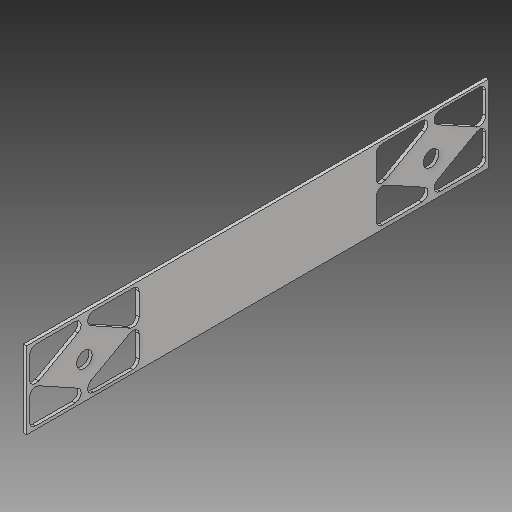
# Autodesk Inventor part: R-SideV1
Saved by Autodesk Inventor 2019 (Build 230136000, 136)
## iProperties
Created: 2021-09-15
Part Number: R-SideV1
Material: Generic
Document SubType Name: Modeling
Designer: timmy
Density: 1 g/cm^3
Appearance: Default
Author: timmy
Autodesk Inventor part; units mm, degrees
ref_plane "YZ Plane" through (0, 0, 0) normal (1, 0, 0) x (0, 1, 0)
ref_plane "XZ Plane" through (0, 0, 0) normal (0, 1, 0) x (-1, 0, 0)
ref_plane "XY Plane" through (0, 0, 0) normal (0, 0, 1) x (1, 0, 0)
sketch "Sketch1" plane through (0, 0, 0) normal (1, 0, 0) x (0, 1, 0)
  line L0 (0, 0) -> (152.4, 0)
  line L1 (152.4, 0) -> (152.4, -914.4)
  line L2 (152.4, -914.4) -> (0, -914.4)
  line L3 (0, -914.4) -> (0, 0)
  dimension "d0" = 152.4
  dimension "d1" = 914.4
  constraints: 8 end point, 2 parallel, 1 horizontal, 1 perpendicular
  measures "d0" distance of L1.end L2.end
  measures "d1" distance of L0.end L1.end
extrude "Extrusion1" add sketch "Sketch1" along normal blind 6.35
sketch "Sketch2" plane through (6.35, 0, 0) normal (1, 0, 0) x (0, 0, -1)
  line L0 (0, 152.4) -> (0, 0) construction
  line L1 (914.4, 152.4) -> (0, 152.4) construction
  line L2 (0, 152.4) -> (457.2, 152.4) construction
  line L3 (228.6, 152.4) -> (0, 152.4) construction
  line L4 (17.9147, 146.1725) -> (95.9969, 146.1725)
  arc A0 (101.8461, 123.5552) -> (95.9969, 146.1725) centre (95.9969, 134.1075) ccw
  line L5 (101.8461, 123.5552) -> (23.7639, 80.2737)
  arc A1 (5.8497, 90.826) -> (23.7639, 80.2737) centre (17.9147, 90.826) ccw
  line L6 (5.8497, 90.826) -> (5.8497, 134.1075)
  arc A2 (17.9147, 146.1725) -> (5.8497, 134.1075) centre (17.9147, 134.1075) ccw
  line L7 (210.6853, 146.1725) -> (132.6031, 146.1725)
  arc A3 (132.6031, 146.1725) -> (126.7539, 123.5552) centre (132.6031, 134.1075) ccw
  line L8 (126.7539, 123.5552) -> (204.8361, 80.2737)
  arc A4 (204.8361, 80.2737) -> (222.7503, 90.826) centre (210.6853, 90.826) ccw
  line L9 (222.7503, 90.826) -> (222.7503, 134.1075)
  arc A5 (222.7503, 134.1075) -> (210.6853, 146.1725) centre (210.6853, 134.1075) ccw
  line L10 (17.9147, 6.2275) -> (95.9969, 6.2275)
  arc A6 (95.9969, 6.2275) -> (101.8461, 28.8448) centre (95.9969, 18.2925) ccw
  line L11 (101.8461, 28.8448) -> (23.7639, 72.1263)
  arc A7 (23.7639, 72.1263) -> (5.8497, 61.574) centre (17.9147, 61.574) ccw
  line L12 (5.8497, 61.574) -> (5.8497, 18.2925)
  arc A8 (5.8497, 18.2925) -> (17.9147, 6.2275) centre (17.9147, 18.2925) ccw
  line L13 (126.7539, 28.8448) -> (204.8361, 72.1263)
  line L14 (210.6853, 6.2275) -> (132.6031, 6.2275)
  line L15 (222.7503, 61.574) -> (222.7503, 18.2925)
  arc A9 (222.7503, 61.574) -> (204.8361, 72.1263) centre (210.6853, 61.574) ccw
  arc A10 (210.6853, 6.2275) -> (222.7503, 18.2925) centre (210.6853, 18.2925) ccw
  arc A11 (126.7539, 28.8448) -> (132.6031, 6.2275) centre (132.6031, 18.2925) ccw
  line L16 (896.5064, 147.907) -> (818.4249, 147.5987)
  arc A12 (818.4249, 147.5987) -> (812.6651, 124.9585) centre (818.4726, 135.5338) ccw
  line L17 (812.6651, 124.9585) -> (890.9175, 81.9857)
  arc A13 (890.9175, 81.9857) -> (908.7899, 92.6086) centre (896.725, 92.561) ccw
  line L18 (908.7899, 92.6086) -> (908.619, 135.8897)
  arc A14 (908.619, 135.8897) -> (896.5064, 147.907) centre (896.5541, 135.8421) ccw
  line L19 (787.7574, 124.8602) -> (709.8468, 81.2707)
  line L20 (703.7374, 147.1459) -> (781.8189, 147.4542)
  line L21 (691.891, 91.7522) -> (691.7201, 135.0333)
  arc A15 (691.891, 91.7522) -> (709.8468, 81.2707) centre (703.9559, 91.7998) ccw
  arc A16 (703.7374, 147.1459) -> (691.7201, 135.0333) centre (703.785, 135.081) ccw
  arc A17 (787.7574, 124.8602) -> (781.8189, 147.4542) centre (781.8665, 135.3893) ccw
  arc A18 (897.059, 7.9631) -> (909.0763, 20.0757) centre (897.0113, 20.028) ccw
  line L22 (897.059, 7.9631) -> (818.9775, 7.6548)
  line L23 (813.039, 30.2488) -> (890.9496, 73.8383)
  arc A19 (813.039, 30.2488) -> (818.9775, 7.6548) centre (818.9298, 19.7197) ccw
  line L24 (908.9054, 63.3568) -> (909.0763, 20.0757)
  arc A20 (908.9054, 63.3568) -> (890.9496, 73.8383) centre (896.8405, 63.3092) ccw
  arc A21 (782.3715, 7.5103) -> (788.1313, 30.1505) centre (782.3238, 19.5752) ccw
  line L25 (704.29, 7.202) -> (782.3715, 7.5103)
  arc A22 (709.8789, 73.1233) -> (692.0065, 62.5004) centre (704.0714, 62.548) ccw
  line L26 (692.0065, 62.5004) -> (692.1774, 19.2192)
  arc A23 (692.1774, 19.2192) -> (704.29, 7.202) centre (704.2423, 19.2669) ccw
  line L27 (788.1313, 30.1505) -> (709.8789, 73.1233)
  circle A24 centre (114.3, 72.0167) radius 15.5575
  circle A25 centre (800.4147, 73.3712) radius 15.5575
  constraints: 52 end point, 48 point on circle, 26 centre point, 2 midpoint, 1 collinear, 1 perpendicular
extrude "Extrusion3" cut sketch "Sketch2" against normal blind 25.4
body "Solid1"
